Autodesk Inventor part; units mm, degrees
(part 2 of 2)
sketch "Top Plate" plane through (0, 0, 0) normal (0, 1, 0) x (-1, 0, 0)
  line L0 (-4.3301, -1.5) -> (65.8, 119.9689)
  line L1 (67.532, 119.9689) -> (137.6621, -1.5)
  line L2 (-3.4641, -3) -> (136.7961, -3)
  circle A0 centre (33.333, 0) radius 1.5
  circle A1 centre (0, 0) radius 1.5
  circle A2 centre (16.6665, 28.8672) radius 1.5
  circle A3 centre (33.333, 57.7344) radius 1.5
  circle A4 centre (49.9995, 28.8672) radius 1.5
  circle A5 centre (66.666, 0) radius 1.5
  circle A6 centre (99.999, 0) radius 1.5
  circle A7 centre (133.332, 0) radius 1.5
  circle A8 centre (116.6655, 28.8672) radius 1.5
  circle A9 centre (99.999, 57.7344) radius 1.5
  circle A10 centre (83.3325, 28.8672) radius 1.5
  circle A11 centre (66.666, 57.7344) radius 1.5
  circle A12 centre (83.3325, 86.6017) radius 1.5
  circle A13 centre (49.9995, 86.6017) radius 1.5
  circle A14 centre (66.666, 115.4689) radius 1.5
  arc A15 (67.532, 119.9689) -> (65.8, 119.9689) centre (66.666, 119.4689) ccw
  arc A16 (136.7961, -3) -> (137.6621, -1.5) centre (136.7961, -2) ccw
  arc A17 (-4.3301, -1.5) -> (-3.4641, -3) centre (-3.4641, -2) ccw
  line L3 (0, 0) -> (-14.4563, -8.3464) construction
  line L4 (133.332, 0) -> (144.2364, -6.2956) construction
  line L5 (27.8865, 48.3008) -> (27.8865, 48.3008)
  line L6 (108.6655, 28.8672) -> (113.6655, 28.8672) construction
  line L7 (98.999, 38.3008) -> (99.999, 38.3008)
  line L8 (0, 0) -> (16.6665, 28.8672) construction
  line L9 (16.6665, 28.8672) -> (33.333, 0) construction
  line L10 (33.333, 0) -> (0, 0) construction
  line L11 (33.333, 0) -> (8.3333, 14.4336) construction
  line L12 (0, 0) -> (24.9998, 14.4336) construction
  line L13 (16.6665, 28.8672) -> (16.6665, 0) construction
  line L14 (0, 14.4336) -> (33.333, 14.4336) construction
  line L15 (0, 19.4336) -> (33.333, 19.4336) construction
  line L16 (0, 9.4336) -> (33.333, 9.4336) construction
  line L17 (16.6665, 19.4336) -> (16.6665, 14.4336) construction
  line L18 (16.6665, 14.4336) -> (16.6665, 9.4336) construction
  circle A18 centre (16.6665, 14.4336) radius 2.5
  circle A19 centre (16.6665, 14.4336) radius 14.4336 construction
  circle A20 centre (6.7821, 3.9156) radius 2.5
  circle A21 centre (26.5509, 3.9156) radius 2.5
  circle A22 centre (16.6665, 14.4336) radius 10 construction
  circle A23 centre (16.6665, 4.4336) radius 2
  circle A24 centre (16.6665, 14.4336) radius 7.5 construction
  circle A25 centre (11.0763, 9.4336) radius 1.5
  circle A26 centre (22.2567, 9.4336) radius 1.5
  circle A27 centre (16.6665, 9.4336) radius 1
  circle A28 centre (16.6665, 21.9336) radius 1.5
  circle A29 centre (16.6665, 14.4336) radius 5 construction
  line L19 (5.4465, 9.4336) -> (22.2567, 19.4336) construction
  line L20 (27.8865, 9.4336) -> (11.0763, 19.4336) construction
  circle A30 centre (20.046, 18.1186) radius 1
  circle A31 centre (13.287, 18.1186) radius 1
  circle A32 centre (16.6665, 14.4336) radius 12.5 construction
  circle A33 centre (21.5432, 2.9241) radius 1.25
  circle A34 centre (11.7898, 2.9241) radius 1.25
  line L21 (16.6665, 4.4336) -> (21.5432, 2.9241) construction
  line L22 (21.5432, 2.9241) -> (26.5509, 3.9156) construction
  line L23 (6.7821, 3.9156) -> (11.7898, 2.9241) construction
  line L24 (11.7898, 2.9241) -> (16.6665, 4.4336) construction
  circle A35 centre (0, 0) radius 2.75 construction
  circle A36 centre (33.333, 0) radius 2.75 construction
  circle A37 centre (16.6665, 28.8672) radius 2.75 construction
  line L25 (33.333, 0) -> (49.9995, 28.8672) construction
  line L26 (49.9995, 28.8672) -> (66.666, 0) construction
  line L27 (66.666, 0) -> (33.333, 0) construction
  line L28 (66.666, 0) -> (41.6663, 14.4336) construction
  line L29 (33.333, 0) -> (58.3328, 14.4336) construction
  line L30 (49.9995, 28.8672) -> (49.9995, 0) construction
  line L31 (33.333, 14.4336) -> (66.666, 14.4336) construction
  line L32 (33.333, 19.4336) -> (66.666, 19.4336) construction
  line L33 (33.333, 9.4336) -> (66.666, 9.4336) construction
  line L34 (49.9995, 19.4336) -> (49.9995, 14.4336) construction
  line L35 (49.9995, 14.4336) -> (49.9995, 9.4336) construction
  circle A38 centre (49.9995, 14.4336) radius 2.5
  circle A39 centre (49.9995, 14.4336) radius 14.4336 construction
  circle A40 centre (40.1151, 3.9156) radius 2.5
  circle A41 centre (59.8839, 3.9156) radius 2.5
  circle A42 centre (49.9995, 14.4336) radius 10 construction
  circle A43 centre (49.9995, 4.4336) radius 2
  circle A44 centre (49.9995, 14.4336) radius 7.5 construction
  circle A45 centre (44.4093, 9.4336) radius 1.5
  circle A46 centre (55.5897, 9.4336) radius 1.5
  circle A47 centre (49.9995, 9.4336) radius 1
  circle A48 centre (49.9995, 21.9336) radius 1.5
  circle A49 centre (49.9995, 14.4336) radius 5 construction
  line L36 (38.7795, 9.4336) -> (55.5897, 19.4336) construction
  line L37 (61.2195, 9.4336) -> (44.4093, 19.4336) construction
  circle A50 centre (53.379, 18.1186) radius 1
  circle A51 centre (46.62, 18.1186) radius 1
  circle A52 centre (49.9995, 14.4336) radius 12.5 construction
  circle A53 centre (54.8762, 2.9241) radius 1.25
  circle A54 centre (45.1228, 2.9241) radius 1.25
  line L38 (49.9995, 4.4336) -> (54.8762, 2.9241) construction
  line L39 (54.8762, 2.9241) -> (59.8839, 3.9156) construction
  line L40 (40.1151, 3.9156) -> (45.1228, 2.9241) construction
  line L41 (45.1228, 2.9241) -> (49.9995, 4.4336) construction
  circle A55 centre (33.333, 0) radius 2.75 construction
  circle A56 centre (66.666, 0) radius 2.75 construction
  circle A57 centre (49.9995, 28.8672) radius 2.75 construction
  line L42 (49.9995, 28.8672) -> (33.333, 0) construction
  line L43 (33.333, 0) -> (16.6665, 28.8672) construction
  line L44 (16.6665, 28.8672) -> (49.9995, 28.8672) construction
  line L45 (16.6665, 28.8672) -> (41.6663, 14.4336) construction
  line L46 (49.9995, 28.8672) -> (24.9998, 14.4336) construction
  line L47 (33.333, 0) -> (33.333, 28.8672) construction
  line L48 (49.9995, 14.4336) -> (16.6665, 14.4336) construction
  line L49 (49.9995, 9.4336) -> (16.6665, 9.4336) construction
  line L50 (49.9995, 19.4336) -> (16.6665, 19.4336) construction
  line L51 (33.333, 9.4336) -> (33.333, 14.4336) construction
  line L52 (33.333, 14.4336) -> (33.333, 19.4336) construction
  circle A58 centre (33.333, 14.4336) radius 2.5
  circle A59 centre (33.333, 14.4336) radius 14.4336 construction
  circle A60 centre (43.2174, 24.9516) radius 2.5
  circle A61 centre (23.4486, 24.9516) radius 2.5
  circle A62 centre (33.333, 14.4336) radius 10 construction
  circle A63 centre (33.333, 24.4336) radius 2
  circle A64 centre (33.333, 14.4336) radius 7.5 construction
  circle A65 centre (38.9232, 19.4336) radius 1.5
  circle A66 centre (27.7428, 19.4336) radius 1.5
  circle A67 centre (33.333, 19.4336) radius 1
  circle A68 centre (33.333, 6.9336) radius 1.5
  circle A69 centre (33.333, 14.4336) radius 5 construction
  line L53 (44.553, 19.4336) -> (27.7428, 9.4336) construction
  line L54 (22.113, 19.4336) -> (38.9232, 9.4336) construction
  circle A70 centre (29.9535, 10.7487) radius 1
  circle A71 centre (36.7125, 10.7487) radius 1
  circle A72 centre (33.333, 14.4336) radius 12.5 construction
  circle A73 centre (28.4563, 25.9431) radius 1.25
  circle A74 centre (38.2097, 25.9431) radius 1.25
  line L55 (33.333, 24.4336) -> (28.4563, 25.9431) construction
  line L56 (28.4563, 25.9431) -> (23.4486, 24.9516) construction
  line L57 (43.2174, 24.9516) -> (38.2097, 25.9431) construction
  line L58 (38.2097, 25.9431) -> (33.333, 24.4336) construction
  circle A75 centre (49.9995, 28.8672) radius 2.75 construction
  circle A76 centre (16.6665, 28.8672) radius 2.75 construction
  circle A77 centre (33.333, 0) radius 2.75 construction
  line L59 (83.3325, 28.8672) -> (66.666, 0) construction
  line L60 (66.666, 0) -> (49.9995, 28.8672) construction
  line L61 (49.9995, 28.8672) -> (83.3325, 28.8672) construction
  line L62 (49.9995, 28.8672) -> (74.9993, 14.4336) construction
  line L63 (83.3325, 28.8672) -> (58.3328, 14.4336) construction
  line L64 (66.666, 0) -> (66.666, 28.8672) construction
  line L65 (83.3325, 14.4336) -> (49.9995, 14.4336) construction
  line L66 (83.3325, 9.4336) -> (49.9995, 9.4336) construction
  line L67 (83.3325, 19.4336) -> (49.9995, 19.4336) construction
  line L68 (66.666, 9.4336) -> (66.666, 14.4336) construction
  line L69 (66.666, 14.4336) -> (66.666, 19.4336) construction
  circle A78 centre (66.666, 14.4336) radius 2.5
  circle A79 centre (66.666, 14.4336) radius 14.4336 construction
  circle A80 centre (76.5504, 24.9516) radius 2.5
  circle A81 centre (56.7816, 24.9516) radius 2.5
  circle A82 centre (66.666, 14.4336) radius 10 construction
  circle A83 centre (66.666, 24.4336) radius 2
  circle A84 centre (66.666, 14.4336) radius 7.5 construction
  circle A85 centre (72.2562, 19.4336) radius 1.5
  circle A86 centre (61.0758, 19.4336) radius 1.5
  circle A87 centre (66.666, 19.4336) radius 1
  circle A88 centre (66.666, 6.9336) radius 1.5
  circle A89 centre (66.666, 14.4336) radius 5 construction
  line L70 (77.886, 19.4336) -> (61.0758, 9.4336) construction
  line L71 (55.446, 19.4336) -> (72.2562, 9.4336) construction
  circle A90 centre (63.2865, 10.7487) radius 1
  circle A91 centre (70.0455, 10.7487) radius 1
  circle A92 centre (66.666, 14.4336) radius 12.5 construction
  circle A93 centre (61.7893, 25.9431) radius 1.25
  circle A94 centre (71.5427, 25.9431) radius 1.25
  line L72 (66.666, 24.4336) -> (61.7893, 25.9431) construction
  line L73 (61.7893, 25.9431) -> (56.7816, 24.9516) construction
  line L74 (76.5504, 24.9516) -> (71.5427, 25.9431) construction
  line L75 (71.5427, 25.9431) -> (66.666, 24.4336) construction
  circle A95 centre (83.3325, 28.8672) radius 2.75 construction
  circle A96 centre (49.9995, 28.8672) radius 2.75 construction
  circle A97 centre (66.666, 0) radius 2.75 construction
  line L76 (66.666, 0) -> (83.3325, 28.8672) construction
  line L77 (83.3325, 28.8672) -> (99.999, 0) construction
  line L78 (99.999, 0) -> (66.666, 0) construction
  line L79 (99.999, 0) -> (74.9993, 14.4336) construction
  line L80 (66.666, 0) -> (91.6658, 14.4336) construction
  line L81 (83.3325, 28.8672) -> (83.3325, 0) construction
  line L82 (66.666, 14.4336) -> (99.999, 14.4336) construction
  line L83 (66.666, 19.4336) -> (99.999, 19.4336) construction
  line L84 (66.666, 9.4336) -> (99.999, 9.4336) construction
  line L85 (83.3325, 19.4336) -> (83.3325, 14.4336) construction
  line L86 (83.3325, 14.4336) -> (83.3325, 9.4336) construction
  circle A98 centre (83.3325, 14.4336) radius 2.5
  circle A99 centre (83.3325, 14.4336) radius 14.4336 construction
  circle A100 centre (73.4481, 3.9156) radius 2.5
  circle A101 centre (93.2169, 3.9156) radius 2.5
  circle A102 centre (83.3325, 14.4336) radius 10 construction
  circle A103 centre (83.3325, 4.4336) radius 2
  circle A104 centre (83.3325, 14.4336) radius 7.5 construction
  circle A105 centre (77.7423, 9.4336) radius 1.5
  circle A106 centre (88.9227, 9.4336) radius 1.5
  circle A107 centre (83.3325, 9.4336) radius 1
  circle A108 centre (83.3325, 21.9336) radius 1.5
  circle A109 centre (83.3325, 14.4336) radius 5 construction
  line L87 (72.1125, 9.4336) -> (88.9227, 19.4336) construction
  line L88 (94.5525, 9.4336) -> (77.7423, 19.4336) construction
  circle A110 centre (86.712, 18.1186) radius 1
  circle A111 centre (79.953, 18.1186) radius 1
  circle A112 centre (83.3325, 14.4336) radius 12.5 construction
  circle A113 centre (88.2092, 2.9241) radius 1.25
  circle A114 centre (78.4558, 2.9241) radius 1.25
  line L89 (83.3325, 4.4336) -> (88.2092, 2.9241) construction
  line L90 (88.2092, 2.9241) -> (93.2169, 3.9156) construction
  line L91 (73.4481, 3.9156) -> (78.4558, 2.9241) construction
  line L92 (78.4558, 2.9241) -> (83.3325, 4.4336) construction
  circle A115 centre (66.666, 0) radius 2.75 construction
  circle A116 centre (99.999, 0) radius 2.75 construction
  circle A117 centre (83.3325, 28.8672) radius 2.75 construction
  line L93 (99.999, 0) -> (116.6655, 28.8672) construction
  line L94 (116.6655, 28.8672) -> (133.332, 0) construction
  line L95 (133.332, 0) -> (99.999, 0) construction
  line L96 (133.332, 0) -> (108.3323, 14.4336) construction
  line L97 (99.999, 0) -> (124.9988, 14.4336) construction
  line L98 (116.6655, 28.8672) -> (116.6655, 0) construction
  line L99 (99.999, 14.4336) -> (133.332, 14.4336) construction
  line L100 (99.999, 19.4336) -> (133.332, 19.4336) construction
  line L101 (99.999, 9.4336) -> (133.332, 9.4336) construction
  line L102 (116.6655, 19.4336) -> (116.6655, 14.4336) construction
  line L103 (116.6655, 14.4336) -> (116.6655, 9.4336) construction
  circle A118 centre (116.6655, 14.4336) radius 2.5
  circle A119 centre (116.6655, 14.4336) radius 14.4336 construction
  circle A120 centre (106.7811, 3.9156) radius 2.5
  circle A121 centre (126.5499, 3.9156) radius 2.5
  circle A122 centre (116.6655, 14.4336) radius 10 construction
  circle A123 centre (116.6655, 4.4336) radius 2
  circle A124 centre (116.6655, 14.4336) radius 7.5 construction
  circle A125 centre (111.0753, 9.4336) radius 1.5
  circle A126 centre (122.2557, 9.4336) radius 1.5
  circle A127 centre (116.6655, 9.4336) radius 1
  circle A128 centre (116.6655, 21.9336) radius 1.5
  circle A129 centre (116.6655, 14.4336) radius 5 construction
  line L104 (105.4455, 9.4336) -> (122.2557, 19.4336) construction
  line L105 (127.8855, 9.4336) -> (111.0753, 19.4336) construction
  circle A130 centre (120.045, 18.1186) radius 1
  circle A131 centre (113.286, 18.1186) radius 1
  circle A132 centre (116.6655, 14.4336) radius 12.5 construction
  circle A133 centre (121.5422, 2.9241) radius 1.25
  circle A134 centre (111.7888, 2.9241) radius 1.25
  line L106 (116.6655, 4.4336) -> (121.5422, 2.9241) construction
  line L107 (121.5422, 2.9241) -> (126.5499, 3.9156) construction
  line L108 (106.7811, 3.9156) -> (111.7888, 2.9241) construction
  line L109 (111.7888, 2.9241) -> (116.6655, 4.4336) construction
  circle A135 centre (99.999, 0) radius 2.75 construction
  circle A136 centre (133.332, 0) radius 2.75 construction
  circle A137 centre (116.6655, 28.8672) radius 2.75 construction
  line L110 (116.6655, 28.8672) -> (99.999, 0) construction
  line L111 (99.999, 0) -> (83.3325, 28.8672) construction
  line L112 (83.3325, 28.8672) -> (116.6655, 28.8672) construction
  line L113 (83.3325, 28.8672) -> (108.3323, 14.4336) construction
  line L114 (116.6655, 28.8672) -> (91.6658, 14.4336) construction
  line L115 (99.999, 0) -> (99.999, 28.8672) construction
  line L116 (116.6655, 14.4336) -> (83.3325, 14.4336) construction
  line L117 (116.6655, 9.4336) -> (83.3325, 9.4336) construction
  line L118 (116.6655, 19.4336) -> (83.3325, 19.4336) construction
  line L119 (99.999, 9.4336) -> (99.999, 14.4336) construction
  line L120 (99.999, 14.4336) -> (99.999, 19.4336) construction
  circle A138 centre (99.999, 14.4336) radius 2.5
  circle A139 centre (99.999, 14.4336) radius 14.4336 construction
  circle A140 centre (109.8834, 24.9516) radius 2.5
  circle A141 centre (90.1146, 24.9516) radius 2.5
  circle A142 centre (99.999, 14.4336) radius 10 construction
  circle A143 centre (99.999, 24.4336) radius 2
  circle A144 centre (99.999, 14.4336) radius 7.5 construction
  circle A145 centre (105.5892, 19.4336) radius 1.5
  circle A146 centre (94.4088, 19.4336) radius 1.5
  circle A147 centre (99.999, 19.4336) radius 1
  circle A148 centre (99.999, 6.9336) radius 1.5
  circle A149 centre (99.999, 14.4336) radius 5 construction
  line L121 (111.219, 19.4336) -> (94.4088, 9.4336) construction
  line L122 (88.779, 19.4336) -> (105.5892, 9.4336) construction
  circle A150 centre (96.6195, 10.7487) radius 1
  circle A151 centre (103.3785, 10.7487) radius 1
  circle A152 centre (99.999, 14.4336) radius 12.5 construction
  circle A153 centre (95.1223, 25.9431) radius 1.25
  circle A154 centre (104.8757, 25.9431) radius 1.25
  line L123 (99.999, 24.4336) -> (95.1223, 25.9431) construction
  line L124 (95.1223, 25.9431) -> (90.1146, 24.9516) construction
  line L125 (109.8834, 24.9516) -> (104.8757, 25.9431) construction
  line L126 (104.8757, 25.9431) -> (99.999, 24.4336) construction
  circle A155 centre (116.6655, 28.8672) radius 2.75 construction
  circle A156 centre (83.3325, 28.8672) radius 2.75 construction
  circle A157 centre (99.999, 0) radius 2.75 construction
  line L127 (16.6665, 28.8672) -> (33.333, 57.7344) construction
  line L128 (33.333, 57.7344) -> (49.9995, 28.8672) construction
  line L129 (49.9995, 28.8672) -> (16.6665, 28.8672) construction
  line L130 (49.9995, 28.8672) -> (24.9998, 43.3008) construction
  line L131 (16.6665, 28.8672) -> (41.6663, 43.3008) construction
  line L132 (33.333, 57.7344) -> (33.333, 28.8672) construction
  line L133 (16.6665, 43.3008) -> (49.9995, 43.3008) construction
  line L134 (16.6665, 48.3008) -> (49.9995, 48.3008) construction
  line L135 (16.6665, 38.3008) -> (49.9995, 38.3008) construction
  line L136 (33.333, 48.3008) -> (33.333, 43.3008) construction
  line L137 (33.333, 43.3008) -> (33.333, 38.3008) construction
  circle A158 centre (33.333, 43.3008) radius 2.5
  circle A159 centre (33.333, 43.3008) radius 14.4336 construction
  circle A160 centre (23.4486, 32.7829) radius 2.5
  circle A161 centre (43.2174, 32.7829) radius 2.5
  circle A162 centre (33.333, 43.3008) radius 10 construction
  circle A163 centre (33.333, 33.3008) radius 2
  circle A164 centre (33.333, 43.3008) radius 7.5 construction
  circle A165 centre (27.7428, 38.3008) radius 1.5
  circle A166 centre (38.9232, 38.3008) radius 1.5
  circle A167 centre (33.333, 38.3008) radius 1
  circle A168 centre (33.333, 50.8008) radius 1.5
  circle A169 centre (33.333, 43.3008) radius 5 construction
  line L138 (22.113, 38.3008) -> (38.9232, 48.3008) construction
  line L139 (44.553, 38.3008) -> (27.7428, 48.3008) construction
  circle A170 centre (36.7125, 46.9858) radius 1
  circle A171 centre (29.9535, 46.9858) radius 1
  circle A172 centre (33.333, 43.3008) radius 12.5 construction
  circle A173 centre (38.2097, 31.7914) radius 1.25
  circle A174 centre (28.4563, 31.7914) radius 1.25
  line L140 (33.333, 33.3008) -> (38.2097, 31.7914) construction
  line L141 (38.2097, 31.7914) -> (43.2174, 32.7829) construction
  line L142 (23.4486, 32.7829) -> (28.4563, 31.7914) construction
  line L143 (28.4563, 31.7914) -> (33.333, 33.3008) construction
  circle A175 centre (16.6665, 28.8672) radius 2.75 construction
  circle A176 centre (49.9995, 28.8672) radius 2.75 construction
  circle A177 centre (33.333, 57.7344) radius 2.75 construction
  line L144 (33.333, 57.7344) -> (49.9995, 86.6017) construction
  line L145 (49.9995, 86.6017) -> (66.666, 57.7344) construction
  line L146 (66.666, 57.7344) -> (33.333, 57.7344) construction
  line L147 (66.666, 57.7344) -> (41.6663, 72.1681) construction
  line L148 (33.333, 57.7344) -> (58.3328, 72.1681) construction
  line L149 (49.9995, 86.6017) -> (49.9995, 57.7344) construction
  line L150 (33.333, 72.1681) -> (66.666, 72.1681) construction
  line L151 (33.333, 77.1681) -> (66.666, 77.1681) construction
  line L152 (33.333, 67.1681) -> (66.666, 67.1681) construction
  line L153 (49.9995, 77.1681) -> (49.9995, 72.1681) construction
  line L154 (49.9995, 72.1681) -> (49.9995, 67.1681) construction
  circle A178 centre (49.9995, 72.1681) radius 2.5
  circle A179 centre (49.9995, 72.1681) radius 14.4336 construction
  circle A180 centre (40.1151, 61.6501) radius 2.5
  circle A181 centre (59.8839, 61.6501) radius 2.5
  circle A182 centre (49.9995, 72.1681) radius 10 construction
  circle A183 centre (49.9995, 62.1681) radius 2
  circle A184 centre (49.9995, 72.1681) radius 7.5 construction
  circle A185 centre (44.4093, 67.1681) radius 1.5
  circle A186 centre (55.5897, 67.1681) radius 1.5
  circle A187 centre (49.9995, 67.1681) radius 1
  circle A188 centre (49.9995, 79.6681) radius 1.5
  circle A189 centre (49.9995, 72.1681) radius 5 construction
  line L155 (38.7795, 67.1681) -> (55.5897, 77.1681) construction
  line L156 (61.2195, 67.1681) -> (44.4093, 77.1681) construction
  circle A190 centre (53.379, 75.853) radius 1
  circle A191 centre (46.62, 75.853) radius 1
  circle A192 centre (49.9995, 72.1681) radius 12.5 construction
  circle A193 centre (54.8762, 60.6586) radius 1.25
  circle A194 centre (45.1228, 60.6586) radius 1.25
  line L157 (49.9995, 62.1681) -> (54.8762, 60.6586) construction
  line L158 (54.8762, 60.6586) -> (59.8839, 61.6501) construction
  line L159 (40.1151, 61.6501) -> (45.1228, 60.6586) construction
  line L160 (45.1228, 60.6586) -> (49.9995, 62.1681) construction
  circle A195 centre (33.333, 57.7344) radius 2.75 construction
  circle A196 centre (66.666, 57.7344) radius 2.75 construction
  circle A197 centre (49.9995, 86.6017) radius 2.75 construction
  line L161 (49.9995, 86.6017) -> (66.666, 115.4689) construction
  line L162 (66.666, 115.4689) -> (83.3325, 86.6017) construction
  line L163 (83.3325, 86.6017) -> (49.9995, 86.6017) construction
  line L164 (83.3325, 86.6017) -> (58.3328, 101.0353) construction
  line L165 (49.9995, 86.6017) -> (74.9993, 101.0353) construction
  line L166 (66.666, 115.4689) -> (66.666, 86.6017) construction
  line L167 (49.9995, 101.0353) -> (83.3325, 101.0353) construction
  line L168 (49.9995, 106.0353) -> (83.3325, 106.0353) construction
  line L169 (49.9995, 96.0353) -> (83.3325, 96.0353) construction
  line L170 (66.666, 106.0353) -> (66.666, 101.0353) construction
  line L171 (66.666, 101.0353) -> (66.666, 96.0353) construction
  circle A198 centre (66.666, 101.0353) radius 2.5
  circle A199 centre (66.666, 101.0353) radius 14.4336 construction
  circle A200 centre (56.7816, 90.5173) radius 2.5
  circle A201 centre (76.5504, 90.5173) radius 2.5
  circle A202 centre (66.666, 101.0353) radius 10 construction
  circle A203 centre (66.666, 91.0353) radius 2
  circle A204 centre (66.666, 101.0353) radius 7.5 construction
  circle A205 centre (61.0758, 96.0353) radius 1.5
  circle A206 centre (72.2562, 96.0353) radius 1.5
  circle A207 centre (66.666, 96.0353) radius 1
  circle A208 centre (66.666, 108.5353) radius 1.5
  circle A209 centre (66.666, 101.0353) radius 5 construction
  line L172 (55.446, 96.0353) -> (72.2562, 106.0353) construction
  line L173 (77.886, 96.0353) -> (61.0758, 106.0353) construction
  circle A210 centre (70.0455, 104.7202) radius 1
  circle A211 centre (63.2865, 104.7202) radius 1
  circle A212 centre (66.666, 101.0353) radius 12.5 construction
  circle A213 centre (71.5427, 89.5258) radius 1.25
  circle A214 centre (61.7893, 89.5258) radius 1.25
  line L174 (66.666, 91.0353) -> (71.5427, 89.5258) construction
  line L175 (71.5427, 89.5258) -> (76.5504, 90.5173) construction
  line L176 (56.7816, 90.5173) -> (61.7893, 89.5258) construction
  line L177 (61.7893, 89.5258) -> (66.666, 91.0353) construction
  circle A215 centre (49.9995, 86.6017) radius 2.75 construction
  circle A216 centre (83.3325, 86.6017) radius 2.75 construction
  circle A217 centre (66.666, 115.4689) radius 2.75 construction
  line L178 (66.666, 57.7344) -> (49.9995, 28.8672) construction
  line L179 (49.9995, 28.8672) -> (33.333, 57.7344) construction
  line L180 (33.333, 57.7344) -> (66.666, 57.7344) construction
  line L181 (33.333, 57.7344) -> (58.3328, 43.3008) construction
  line L182 (66.666, 57.7344) -> (41.6663, 43.3008) construction
  line L183 (49.9995, 28.8672) -> (49.9995, 57.7344) construction
  line L184 (66.666, 43.3008) -> (33.333, 43.3008) construction
  line L185 (66.666, 38.3008) -> (33.333, 38.3008) construction
  line L186 (66.666, 48.3008) -> (33.333, 48.3008) construction
  line L187 (49.9995, 38.3008) -> (49.9995, 43.3008) construction
  line L188 (49.9995, 43.3008) -> (49.9995, 48.3008) construction
  circle A218 centre (49.9995, 43.3008) radius 2.5
  circle A219 centre (49.9995, 43.3008) radius 14.4336 construction
  circle A220 centre (59.8839, 53.8188) radius 2.5
  circle A221 centre (40.1151, 53.8188) radius 2.5
  circle A222 centre (49.9995, 43.3008) radius 10 construction
  circle A223 centre (49.9995, 53.3008) radius 2
  circle A224 centre (49.9995, 43.3008) radius 7.5 construction
  circle A225 centre (55.5897, 48.3008) radius 1.5
  circle A226 centre (44.4093, 48.3008) radius 1.5
  circle A227 centre (49.9995, 48.3008) radius 1
  circle A228 centre (49.9995, 35.8008) radius 1.5
  circle A229 centre (49.9995, 43.3008) radius 5 construction
  line L189 (61.2195, 48.3008) -> (44.4093, 38.3008) construction
  line L190 (38.7795, 48.3008) -> (55.5897, 38.3008) construction
  circle A230 centre (46.62, 39.6159) radius 1
  circle A231 centre (53.379, 39.6159) radius 1
  circle A232 centre (49.9995, 43.3008) radius 12.5 construction
  circle A233 centre (45.1228, 54.8103) radius 1.25
  circle A234 centre (54.8762, 54.8103) radius 1.25
  line L191 (49.9995, 53.3008) -> (45.1228, 54.8103) construction
  line L192 (45.1228, 54.8103) -> (40.1151, 53.8188) construction
  line L193 (59.8839, 53.8188) -> (54.8762, 54.8103) construction
  line L194 (54.8762, 54.8103) -> (49.9995, 53.3008) construction
  circle A235 centre (66.666, 57.7344) radius 2.75 construction
  circle A236 centre (33.333, 57.7344) radius 2.75 construction
  circle A237 centre (49.9995, 28.8672) radius 2.75 construction
  line L195 (83.3325, 86.6017) -> (66.666, 57.7344) construction
  line L196 (66.666, 57.7344) -> (49.9995, 86.6017) construction
  line L197 (49.9995, 86.6017) -> (83.3325, 86.6017) construction
  line L198 (49.9995, 86.6017) -> (74.9993, 72.1681) construction
  line L199 (83.3325, 86.6017) -> (58.3328, 72.1681) construction
  line L200 (66.666, 57.7344) -> (66.666, 86.6017) construction
  line L201 (83.3325, 72.1681) -> (49.9995, 72.1681) construction
  line L202 (83.3325, 67.1681) -> (49.9995, 67.1681) construction
  line L203 (83.3325, 77.1681) -> (49.9995, 77.1681) construction
  line L204 (66.666, 67.1681) -> (66.666, 72.1681) construction
  line L205 (66.666, 72.1681) -> (66.666, 77.1681) construction
  circle A238 centre (66.666, 72.1681) radius 2.5
  circle A239 centre (66.666, 72.1681) radius 14.4336 construction
  circle A240 centre (76.5504, 82.686) radius 2.5
  circle A241 centre (56.7816, 82.686) radius 2.5
  circle A242 centre (66.666, 72.1681) radius 10 construction
  circle A243 centre (66.666, 82.1681) radius 2
  circle A244 centre (66.666, 72.1681) radius 7.5 construction
  circle A245 centre (72.2562, 77.1681) radius 1.5
  circle A246 centre (61.0758, 77.1681) radius 1.5
  circle A247 centre (66.666, 77.1681) radius 1
  circle A248 centre (66.666, 64.6681) radius 1.5
  circle A249 centre (66.666, 72.1681) radius 5 construction
  line L206 (77.886, 77.1681) -> (61.0758, 67.1681) construction
  line L207 (55.446, 77.1681) -> (72.2562, 67.1681) construction
  circle A250 centre (63.2865, 68.4831) radius 1
  circle A251 centre (70.0455, 68.4831) radius 1
  circle A252 centre (66.666, 72.1681) radius 12.5 construction
  circle A253 centre (61.7893, 83.6775) radius 1.25
  circle A254 centre (71.5427, 83.6775) radius 1.25
  line L208 (66.666, 82.1681) -> (61.7893, 83.6775) construction
  line L209 (61.7893, 83.6775) -> (56.7816, 82.686) construction
  line L210 (76.5504, 82.686) -> (71.5427, 83.6775) construction
  line L211 (71.5427, 83.6775) -> (66.666, 82.1681) construction
  circle A255 centre (83.3325, 86.6017) radius 2.75 construction
  circle A256 centre (49.9995, 86.6017) radius 2.75 construction
  circle A257 centre (66.666, 57.7344) radius 2.75 construction
  line L212 (66.666, 57.7344) -> (83.3325, 86.6017) construction
  line L213 (83.3325, 86.6017) -> (99.999, 57.7344) construction
  line L214 (99.999, 57.7344) -> (66.666, 57.7344) construction
  line L215 (99.999, 57.7344) -> (74.9993, 72.1681) construction
  line L216 (66.666, 57.7344) -> (91.6658, 72.1681) construction
  line L217 (83.3325, 86.6017) -> (83.3325, 57.7344) construction
  line L218 (66.666, 72.1681) -> (99.999, 72.1681) construction
  line L219 (66.666, 77.1681) -> (99.999, 77.1681) construction
  line L220 (66.666, 67.1681) -> (99.999, 67.1681) construction
  line L221 (83.3325, 77.1681) -> (83.3325, 72.1681) construction
  line L222 (83.3325, 72.1681) -> (83.3325, 67.1681) construction
  circle A258 centre (83.3325, 72.1681) radius 2.5
  circle A259 centre (83.3325, 72.1681) radius 14.4336 construction
  circle A260 centre (73.4481, 61.6501) radius 2.5
  circle A261 centre (93.2169, 61.6501) radius 2.5
  circle A262 centre (83.3325, 72.1681) radius 10 construction
  circle A263 centre (83.3325, 62.1681) radius 2
  circle A264 centre (83.3325, 72.1681) radius 7.5 construction
  circle A265 centre (77.7423, 67.1681) radius 1.5
  circle A266 centre (88.9227, 67.1681) radius 1.5
  circle A267 centre (83.3325, 67.1681) radius 1
  circle A268 centre (83.3325, 79.6681) radius 1.5
  circle A269 centre (83.3325, 72.1681) radius 5 construction
  line L223 (72.1125, 67.1681) -> (88.9227, 77.1681) construction
  line L224 (94.5525, 67.1681) -> (77.7423, 77.1681) construction
  circle A270 centre (86.712, 75.853) radius 1
  circle A271 centre (79.953, 75.853) radius 1
  circle A272 centre (83.3325, 72.1681) radius 12.5 construction
  circle A273 centre (88.2092, 60.6586) radius 1.25
  circle A274 centre (78.4558, 60.6586) radius 1.25
  line L225 (83.3325, 62.1681) -> (88.2092, 60.6586) construction
  line L226 (88.2092, 60.6586) -> (93.2169, 61.6501) construction
  line L227 (73.4481, 61.6501) -> (78.4558, 60.6586) construction
  line L228 (78.4558, 60.6586) -> (83.3325, 62.1681) construction
  circle A275 centre (66.666, 57.7344) radius 2.75 construction
  circle A276 centre (99.999, 57.7344) radius 2.75 construction
  circle A277 centre (83.3325, 86.6017) radius 2.75 construction
  line L229 (49.9995, 28.8672) -> (66.666, 57.7344) construction
  line L230 (66.666, 57.7344) -> (83.3325, 28.8672) construction
  line L231 (83.3325, 28.8672) -> (49.9995, 28.8672) construction
  line L232 (83.3325, 28.8672) -> (58.3328, 43.3008) construction
  line L233 (49.9995, 28.8672) -> (74.9993, 43.3008) construction
  line L234 (66.666, 57.7344) -> (66.666, 28.8672) construction
  line L235 (49.9995, 43.3008) -> (83.3325, 43.3008) construction
  line L236 (49.9995, 48.3008) -> (83.3325, 48.3008) construction
  line L237 (49.9995, 38.3008) -> (83.3325, 38.3008) construction
  line L238 (66.666, 48.3008) -> (66.666, 43.3008) construction
  line L239 (66.666, 43.3008) -> (66.666, 38.3008) construction
  circle A278 centre (66.666, 43.3008) radius 2.5
  circle A279 centre (66.666, 43.3008) radius 14.4336 construction
  circle A280 centre (56.7816, 32.7829) radius 2.5
  circle A281 centre (76.5504, 32.7829) radius 2.5
  circle A282 centre (66.666, 43.3008) radius 10 construction
  circle A283 centre (66.666, 33.3008) radius 2
  circle A284 centre (66.666, 43.3008) radius 7.5 construction
  circle A285 centre (61.0758, 38.3008) radius 1.5
  circle A286 centre (72.2562, 38.3008) radius 1.5
  circle A287 centre (66.666, 38.3008) radius 1
  circle A288 centre (66.666, 50.8008) radius 1.5
  circle A289 centre (66.666, 43.3008) radius 5 construction
  line L240 (55.446, 38.3008) -> (72.2562, 48.3008) construction
  line L241 (77.886, 38.3008) -> (61.0758, 48.3008) construction
  circle A290 centre (70.0455, 46.9858) radius 1
  circle A291 centre (63.2865, 46.9858) radius 1
  circle A292 centre (66.666, 43.3008) radius 12.5 construction
  circle A293 centre (71.5427, 31.7914) radius 1.25
  circle A294 centre (61.7893, 31.7914) radius 1.25
  line L242 (66.666, 33.3008) -> (71.5427, 31.7914) construction
  line L243 (71.5427, 31.7914) -> (76.5504, 32.7829) construction
  line L244 (56.7816, 32.7829) -> (61.7893, 31.7914) construction
  line L245 (61.7893, 31.7914) -> (66.666, 33.3008) construction
  circle A295 centre (49.9995, 28.8672) radius 2.75 construction
  circle A296 centre (83.3325, 28.8672) radius 2.75 construction
  circle A297 centre (66.666, 57.7344) radius 2.75 construction
  line L246 (83.3325, 28.8672) -> (99.999, 57.7344) construction
  line L247 (99.999, 57.7344) -> (116.6655, 28.8672) construction
  line L248 (116.6655, 28.8672) -> (83.3325, 28.8672) construction
  line L249 (116.6655, 28.8672) -> (91.6658, 43.3008) construction
  line L250 (83.3325, 28.8672) -> (108.3323, 43.3008) construction
  line L251 (99.999, 57.7344) -> (99.999, 28.8672) construction
  line L252 (83.3325, 43.3008) -> (116.6655, 43.3008) construction
  line L253 (83.3325, 48.3008) -> (116.6655, 48.3008) construction
  line L254 (83.3325, 38.3008) -> (116.6655, 38.3008) construction
  line L255 (99.999, 48.3008) -> (99.999, 43.3008) construction
  line L256 (99.999, 43.3008) -> (99.999, 38.3008) construction
  circle A298 centre (99.999, 43.3008) radius 2.5
  circle A299 centre (99.999, 43.3008) radius 14.4336 construction
  circle A300 centre (90.1146, 32.7829) radius 2.5
  circle A301 centre (109.8834, 32.7829) radius 2.5
  circle A302 centre (99.999, 43.3008) radius 10 construction
  circle A303 centre (99.999, 33.3008) radius 2
  circle A304 centre (99.999, 43.3008) radius 7.5 construction
  circle A305 centre (94.4088, 38.3008) radius 1.5
  circle A306 centre (105.5892, 38.3008) radius 1.5
  circle A307 centre (99.999, 38.3008) radius 1
  circle A308 centre (99.999, 50.8008) radius 1.5
  circle A309 centre (99.999, 43.3008) radius 5 construction
  line L257 (88.779, 38.3008) -> (105.5892, 48.3008) construction
  line L258 (111.219, 38.3008) -> (94.4088, 48.3008) construction
  circle A310 centre (103.3785, 46.9858) radius 1
  circle A311 centre (96.6195, 46.9858) radius 1
  circle A312 centre (99.999, 43.3008) radius 12.5 construction
  circle A313 centre (104.8757, 31.7914) radius 1.25
  circle A314 centre (95.1223, 31.7914) radius 1.25
  line L259 (99.999, 33.3008) -> (104.8757, 31.7914) construction
  line L260 (104.8757, 31.7914) -> (109.8834, 32.7829) construction
  line L261 (90.1146, 32.7829) -> (95.1223, 31.7914) construction
  line L262 (95.1223, 31.7914) -> (99.999, 33.3008) construction
  circle A315 centre (83.3325, 28.8672) radius 2.75 construction
  circle A316 centre (116.6655, 28.8672) radius 2.75 construction
  circle A317 centre (99.999, 57.7344) radius 2.75 construction
  line L263 (99.999, 57.7344) -> (83.3325, 28.8672) construction
  line L264 (83.3325, 28.8672) -> (66.666, 57.7344) construction
  line L265 (66.666, 57.7344) -> (99.999, 57.7344) construction
  line L266 (66.666, 57.7344) -> (91.6658, 43.3008) construction
  line L267 (99.999, 57.7344) -> (74.9993, 43.3008) construction
  line L268 (83.3325, 28.8672) -> (83.3325, 57.7344) construction
  line L269 (99.999, 43.3008) -> (66.666, 43.3008) construction
  line L270 (99.999, 38.3008) -> (66.666, 38.3008) construction
  line L271 (99.999, 48.3008) -> (66.666, 48.3008) construction
  line L272 (83.3325, 38.3008) -> (83.3325, 43.3008) construction
  line L273 (83.3325, 43.3008) -> (83.3325, 48.3008) construction
  circle A318 centre (83.3325, 43.3008) radius 2.5
  circle A319 centre (83.3325, 43.3008) radius 14.4336 construction
  circle A320 centre (93.2169, 53.8188) radius 2.5
  circle A321 centre (73.4481, 53.8188) radius 2.5
  circle A322 centre (83.3325, 43.3008) radius 10 construction
  circle A323 centre (83.3325, 53.3008) radius 2
  circle A324 centre (83.3325, 43.3008) radius 7.5 construction
  circle A325 centre (88.9227, 48.3008) radius 1.5
  circle A326 centre (77.7423, 48.3008) radius 1.5
  circle A327 centre (83.3325, 48.3008) radius 1
  circle A328 centre (83.3325, 35.8008) radius 1.5
  circle A329 centre (83.3325, 43.3008) radius 5 construction
  line L274 (94.5525, 48.3008) -> (77.7423, 38.3008) construction
  line L275 (72.1125, 48.3008) -> (88.9227, 38.3008) construction
  circle A330 centre (79.953, 39.6159) radius 1
  circle A331 centre (86.712, 39.6159) radius 1
  circle A332 centre (83.3325, 43.3008) radius 12.5 construction
  circle A333 centre (78.4558, 54.8103) radius 1.25
  circle A334 centre (88.2092, 54.8103) radius 1.25
  line L276 (83.3325, 53.3008) -> (78.4558, 54.8103) construction
  line L277 (78.4558, 54.8103) -> (73.4481, 53.8188) construction
  line L278 (93.2169, 53.8188) -> (88.2092, 54.8103) construction
  line L279 (88.2092, 54.8103) -> (83.3325, 53.3008) construction
  circle A335 centre (99.999, 57.7344) radius 2.75 construction
  circle A336 centre (66.666, 57.7344) radius 2.75 construction
  circle A337 centre (83.3325, 28.8672) radius 2.75 construction
  dimension "d25" = 3
  dimension "d35" = 3
  dimension "d36" = 1
  constraints: 18 centre point, 16 end point, 16 equal radius, 6 point on circle, 6 tangent, 3 horizontal, 2 point on line, 26 other
  measures "d25" diameter of A0
  measures "d35" distance from line of L2 A6.centre
  measures "d36" radius of A16
extrude "Extrusion4" add sketch "Top Plate" along normal blind 3
body "Solid4"
